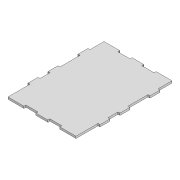
# Autodesk Inventor part: Lat 1
Saved by Autodesk Inventor 2022 (Build 260153000, 153)
## iProperties
Created: 2022-06-21
Part Number: Lat 1
Material: Generic
Document SubType Name: Modeling
Designer: ADMIN
Density: 1 g/cm^3
Appearance: Default
Author: ADMIN
Autodesk Inventor part; units mm, degrees
ref_plane "YZ Plane" through (0, 0, 0) normal (1, 0, 0) x (0, 1, 0)
ref_plane "XZ Plane" through (0, 0, 0) normal (0, 1, 0) x (-1, 0, 0)
ref_plane "XY Plane" through (0, 0, 0) normal (0, 0, 1) x (1, 0, 0)
sketch "Sketch1" plane through (0, 0, 0) normal (0, 1, 0) x (-1, 0, 0)
  line L0 (4.0305, 15.695) -> (174.0305, 15.695)
  line L1 (174.0305, 15.695) -> (174.0305, -224.305)
  line L2 (174.0305, -224.305) -> (4.0305, -224.305)
  line L3 (4.0305, -224.305) -> (4.0305, 15.695)
  line L4 (174.0305, -39.305) -> (169.0305, -39.305)
  line L5 (169.0305, -39.305) -> (169.0305, -64.305)
  line L6 (169.0305, -64.305) -> (174.0305, -64.305)
  line L7 (174.0305, -64.305) -> (174.0305, -39.305)
  line L8 (174.0305, -89.305) -> (169.0305, -89.305)
  line L9 (169.0305, -89.305) -> (169.0305, -114.305)
  line L10 (169.0305, -114.305) -> (174.0305, -114.305)
  line L11 (174.0305, -114.305) -> (174.0305, -89.305)
  line L12 (174.0305, -164.305) -> (169.0305, -164.305)
  line L13 (169.0305, -164.305) -> (169.0305, -189.305)
  line L14 (169.0305, -189.305) -> (174.0305, -189.305)
  line L15 (174.0305, -189.305) -> (174.0305, -164.305)
  line L16 (89.0305, 15.695) -> (89.0305, -224.305)
  line L17 (4.0305, -39.305) -> (9.0305, -39.305)
  line L18 (9.0305, -39.305) -> (9.0305, -64.305)
  line L19 (9.0305, -64.305) -> (4.0305, -64.305)
  line L20 (4.0305, -89.305) -> (9.0305, -89.305)
  line L21 (9.0305, -89.305) -> (9.0305, -114.305)
  line L22 (9.0305, -114.305) -> (4.0305, -114.305)
  line L23 (4.0305, -164.305) -> (9.0305, -164.305)
  line L24 (9.0305, -164.305) -> (9.0305, -189.305)
  line L25 (9.0305, -189.305) -> (4.0305, -189.305)
  line L26 (134.0305, 15.695) -> (104.0305, 15.695)
  line L27 (104.0305, 15.695) -> (104.0305, 10.695)
  line L28 (104.0305, 10.695) -> (134.0305, 10.695)
  line L29 (134.0305, 10.695) -> (134.0305, 15.695)
  line L30 (74.0305, 15.695) -> (44.0305, 15.695)
  line L31 (44.0305, 15.695) -> (44.0305, 10.695)
  line L32 (44.0305, 10.695) -> (74.0305, 10.695)
  line L33 (74.0305, 10.695) -> (74.0305, 15.695)
  line L34 (134.0305, -224.305) -> (104.0305, -224.305)
  line L35 (104.0305, -224.305) -> (104.0305, -219.305)
  line L36 (104.0305, -219.305) -> (134.0305, -219.305)
  line L37 (134.0305, -219.305) -> (134.0305, -224.305)
  line L38 (74.0305, -224.305) -> (44.0305, -224.305)
  line L39 (44.0305, -224.305) -> (44.0305, -219.305)
  line L40 (44.0305, -219.305) -> (74.0305, -219.305)
  line L41 (74.0305, -219.305) -> (74.0305, -224.305)
  line L42 (9.0305, -39.305) -> (-0.9695, -39.305)
  line L43 (-0.9695, -39.305) -> (-0.9695, -64.305)
  line L44 (-0.9695, -64.305) -> (9.0305, -64.305)
  line L45 (9.0305, -64.305) -> (9.0305, -39.305)
  line L46 (9.0305, -89.305) -> (-0.9695, -89.305)
  line L47 (-0.9695, -89.305) -> (-0.9695, -114.305)
  line L48 (-0.9695, -114.305) -> (9.0305, -114.305)
  line L49 (9.0305, -114.305) -> (9.0305, -89.305)
  line L50 (9.0305, -164.305) -> (-0.9695, -164.305)
  line L51 (-0.9695, -164.305) -> (-0.9695, -189.305)
  line L52 (-0.9695, -189.305) -> (9.0305, -189.305)
  line L53 (9.0305, -189.305) -> (9.0305, -164.305)
  line L54 (169.0305, -39.305) -> (179.0305, -39.305)
  line L55 (179.0305, -39.305) -> (179.0305, -64.305)
  line L56 (179.0305, -64.305) -> (169.0305, -64.305)
  line L57 (169.0305, -89.305) -> (179.0305, -89.305)
  line L58 (179.0305, -89.305) -> (179.0305, -114.305)
  line L59 (179.0305, -114.305) -> (169.0305, -114.305)
  line L60 (169.0305, -164.305) -> (179.0305, -164.305)
  line L61 (179.0305, -164.305) -> (179.0305, -189.305)
  line L62 (179.0305, -189.305) -> (169.0305, -189.305)
  point P0 (0, 0)
  dimension "d0" = 170
  dimension "d1" = 240
  dimension "d2" = 5
  dimension "d3" = 25
  dimension "d4" = 5
  dimension "d5" = 25
  dimension "d6" = 5
  dimension "d7" = 25
  dimension "d8" = 35
  dimension "d9" = 50
  dimension "d10" = 25
  dimension "d11" = 30
  dimension "d12" = 30
  dimension "d13" = 5
  dimension "d14" = 5
  dimension "d15" = 30
  dimension "d16" = 15
  dimension "d17" = 5
  dimension "d20" = 10
  dimension "d21" = 10
  constraints: 126 end point, 22 parallel, 21 symmetric about line, 11 horizontal, 11 perpendicular, 10 point on line, 2 midpoint
  measures "d0" distance of L1.end L2.end
  measures "d1" distance of L0.end L1.end
  measures "d2" distance of L6.end L5.end
  measures "d3" distance of L5.end L4.end
  measures "d4" distance of L10.end L9.end
  measures "d5" distance of L9.end L8.end
  measures "d6" distance of L14.end L13.end
  measures "d7" distance of L13.end L12.end
  measures "d8" distance between parallel lines of L2 L14
  measures "d9" distance between parallel lines of L10 L12
  measures "d10" distance between parallel lines of L6 L8
  measures "d11" distance of L28.end L27.end
  measures "d12" distance of L32.end L31.end
  measures "d13" distance of L31.end L30.end
  measures "d14" distance of L28.end L26.start
  measures "d15" distance between parallel lines of L33 L27
  measures "d16" distance between parallel lines of L16 L27
  measures "d17" distance of L34.end L35.end
  measures "d20" distance of L44.end L43.end
  measures "d21" distance of L48.end L47.end
extrude "Extrusion1" add sketch "Sketch1" along normal blind 5 contours L0 L31 L32 L33 L16 L2 L41 L40 L39 L3 L25 L24 L23 L22 L21 L20 L19 L18 L17 | L17 L18 L19 L3 | L3 L44 L43 L42 | L0 L27 L28 L29 L1 L4 L5 L6 L8 L9 L10 L12 L13 L14 L2 L37 L36 L35 L16 | L20 L21 L22 L3 | L3 L48 L47 L46 | L23 L24 L25 L3 | L3 L52 L51 L50 | L54 L55 L56 L1 | L1 L6 L5 L4 | L14 L13 L12 L1 | L1 L60 L61 L62 | L57 L58 L59 L1 | L1 L10 L9 L8
equation "\"d16\" = 0.5 * d15"
body "Solid1"
